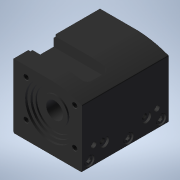
# Autodesk Inventor part: EGC-80-TB-KF___(0_0_Deckel RE)
Saved by Autodesk Inventor 2021 (Build 250183000, 183)
## iProperties
Created: 2026-04-25
Part Number: EGC-80-TB-KF___(0_0_Deckel RE)
Material: Generic
Catalog Web Link: www.3dfindit.com
Description: EGC-RE-TB-Antriebsdeckel RE
Vendor: FESTO
Document SubType Name: Modeling
Designer: psAdmin
Manufacturer: FESTO
Mass: 244.386 g
Surface Area: 426.779 cm^2
Volume: 244.386 cm^3
Density: 1 g/cm^3
Appearance: PSOLRGB-176-176-176
Category: PARTsolutions
Company: FESTO
Title: EGC-80-TB-KF___(0_0_Deckel RE)
Author: Cadenas PARTsolutions
Comments: Antriebsdeckel RE
PSOL_IDENT_0: {$CADENAS_DATA/23d-libs/festo/parts/e/egc/parts/egc_tb_deckel_re.prj},221 {VTYP=3D},{NB=EGC-80-TB-KF
PSOL_IDENT_1: ___(0_0_Deckel RE)},{LINA=EGC-80-TB-KF___(0_0_Deckel RE)},{NN=EGC-RE-TB},{DATE=12.11.2020 08:38:39},
PSOL_IDENT_2: {GEOMDATE=30.04.2020 12:28:00},{VERSION=},{LINEID=30},{WBVAR=ZUBA,ZUBC},{WBNUMERIC=ZUBA,ZUBC}  {NB=E
PSOL_IDENT_3: GC-80-TB-KF___(0_0_Deckel RE)},{LINA=EGC-80-TB-KF___(0_0_Deckel RE)},{KT=DUMMY},{TYP=EGC-80-TB-KF},{
PSOL_IDENT_4: VERS=3.000},{SIZE=80.000},{ZUBA=0},{ZUBC=0},{D1=48},{D2=16},{D3=46.5},{D4=25},{T1=2.1},{T2=27.0},{T4=
PSOL_IDENT_5: 4.00}
NB: EGC-80-TB-KF___(0_0_Deckel RE)
NN: EGC-RE-TB
NT: Antriebsdeckel RE
NBSYN: $TYP.___($ZUBA._$ZUBC._Deckel RE)
LINA: EGC-80-TB-KF___(0_0_Deckel RE)
CATALOG: Festo
TYP: EGC-80-TB-KF
VERS: 3
SIZE: 80
ZUBA: 0
ZUBC: 0
D1: 48
D2: 16
D3: 46.5
D4: 25
T1: 2.1
T2: 27
T4: 4
SUPPLIER: FESTO
ARTICLENO: EGC-80-TB-KF___(0_0_Deckel RE)
BOMINFO: EGC-80-TB-KF___(0_0_Deckel RE)
CREATOR: CADENAS GmbH
Autodesk Inventor part; units mm, degrees
sketch "Sketch_28" plane through (0, 0, 0) normal (0, 0, 1) x (1, 0, 0)
  line L0 (0, 61) -> (0, 0)
  line L1 (0, 0) -> (65, 0)
  line L2 (65, 0) -> (65, 55)
  arc A0 (65, 55) -> (36.5, 61) centre (32.036, -30.8916) ccw
  line L3 (36.5, 61) -> (0, 61)
  constraints: 8 end point, 2 point on circle, 1 centre point
extrude "Extrusion1" add sketch "Sketch_28" along normal blind 82
sketch "Sketch_20" plane through (0, 0, 0) normal (0, 0, 1) x (1, 0, 0)
  line L0 (-2, 5) -> (-2, -1)
  line L1 (-2, -1) -> (66, -1)
  line L2 (66, -1) -> (66, 57)
  line L3 (66, 57) -> (64, 57)
  line L4 (64, 57) -> (64, 55.4781)
  arc A0 (64.4301, 55.2752) -> (64, 55.4781) centre (38.6219, 1.1094) ccw
  arc A1 (65, 54.3725) -> (64.4301, 55.2752) centre (64, 54.3725) ccw
  line L5 (65, 54.3725) -> (65, 1)
  arc A2 (64, 0) -> (65, 1) centre (64, 1) ccw
  line L6 (64, 0) -> (1, 0)
  arc A3 (0, 1) -> (1, 0) centre (1, 1) ccw
  line L7 (0, 1) -> (0, 5)
  line L8 (0, 5) -> (-2, 5)
  constraints: 18 end point, 8 point on circle, 4 centre point
extrude "Extrusion2" cut sketch "Sketch_20" along normal blind 82
sketch "Sketch3" plane through (0, 0, 82) normal (0, 0, 1) x (1, 0, 0)
  point P0 (12, 16.5)
hole "Hole1" at (12, 16.5, 82) direction (0, 0, -1) diameter 4.134 depth 13 tip angle 120 countersink diameter 5 countersink angle 90 thread size "M5x0.8" class "6H" standard "ISO Metric profile"
sketch "Sketch4" plane through (0, 0, 82) normal (0, 0, 1) x (1, 0, 0)
  point P0 (12, 51.5)
hole "Hole2" at (12, 51.5, 82) direction (0, 0, -1) diameter 4.134 depth 13 tip angle 120 countersink diameter 5 countersink angle 90 thread size "M5x0.8" class "6H" standard "ISO Metric profile"
sketch "Sketch5" plane through (0, 0, 0) normal (0, 0, -1) x (-1, 0, 0)
  point P0 (-12, 16.5)
hole "Hole3" at (12, 16.5, 0) direction (0, 0, 1) diameter 4.134 depth 13 tip angle 120 countersink diameter 5 countersink angle 90 thread size "M5x0.8" class "6H" standard "ISO Metric profile"
sketch "Sketch6" plane through (0, 0, 0) normal (0, 0, -1) x (-1, 0, 0)
  point P0 (-12, 51.5)
hole "Hole4" at (12, 51.5, 0) direction (0, 0, 1) diameter 4.134 depth 13 tip angle 120 countersink diameter 5 countersink angle 90 thread size "M5x0.8" class "6H" standard "ISO Metric profile"
sketch "Sketch7" plane through (0, 0, 82) normal (0, 0, 1) x (1, 0, 0)
  point P0 (58, 16.5)
hole "Hole5" at (58, 16.5, 82) direction (0, 0, -1) diameter 4.134 depth 13 tip angle 120 countersink diameter 5 countersink angle 90 thread size "M5x0.8" class "6H" standard "ISO Metric profile"
sketch "Sketch8" plane through (0, 0, 82) normal (0, 0, 1) x (1, 0, 0)
  point P0 (58, 51.5)
hole "Hole6" at (58, 51.5, 82) direction (0, 0, -1) diameter 4.134 depth 13 tip angle 120 countersink diameter 5 countersink angle 90 thread size "M5x0.8" class "6H" standard "ISO Metric profile"
sketch "Sketch9" plane through (0, 0, 0) normal (0, 0, -1) x (-1, 0, 0)
  point P0 (-58, 16.5)
hole "Hole7" at (58, 16.5, 0) direction (0, 0, 1) diameter 4.134 depth 13 tip angle 120 countersink diameter 5 countersink angle 90 thread size "M5x0.8" class "6H" standard "ISO Metric profile"
sketch "Sketch10" plane through (0, 0, 0) normal (0, 0, -1) x (-1, 0, 0)
  point P0 (-58, 51.5)
hole "Hole8" at (58, 51.5, 0) direction (0, 0, 1) diameter 4.134 depth 13 tip angle 120 countersink diameter 5 countersink angle 90 thread size "M5x0.8" class "6H" standard "ISO Metric profile"
sketch "Sketch_13" plane through (0, 0, 0) normal (1, 0, 0) x (0, 1, 0)
  circle A0 centre (55.5, 71) radius 2.85
  constraints: 1 centre point
extrude "Extrusion3" add sketch "Sketch_13" against normal blind 2
sketch "Sketch12" plane through (65, 1, 0) normal (1, 0, 0) x (0, 0, -1)
  point P0 (-71, 16)
hole "Hole9" at (65, 17, 71) direction (-1, 0, 0) diameter 5 depth 3.1
sketch "Sketch13" plane through (65, 1, 0) normal (1, 0, 0) x (0, 0, -1)
  point P0 (-11, 16)
hole "Hole10" at (65, 17, 11) direction (-1, 0, 0) diameter 5 depth 3.1
sketch "Sketch_18" plane through (0, 14.5, 0) normal (0, 1, 0) x (1, 0, 0)
  line L0 (65, -61) -> (50.7066, -61)
  line L1 (50.7066, -61) -> (51.9, -58.933)
  line L2 (51.9, -58.933) -> (62.467, -58.933)
  line L3 (62.467, -58.933) -> (62.9, -58.5)
  line L4 (62.9, -58.5) -> (62.9, -56.5)
  line L5 (62.9, -56.5) -> (65, -56.5)
  line L6 (65, -56.5) -> (65, -61)
  line L7 (65, -61) -> (50.7066, -61)
  constraints: 16 end point
revolve "Revolution1" cut sketch "Sketch_18" angle 360 about axis through (65, 14.5, 61) along (1, 0, 0)
thread "Thread1" size "M5x0.8" class "6H" standard "ISO Metric profile" length 7.567
sketch "Sketch_19" plane through (0, 14.5, 0) normal (0, 1, 0) x (1, 0, 0)
  line L0 (65, -21) -> (50.7066, -21)
  line L1 (50.7066, -21) -> (51.9, -18.933)
  line L2 (51.9, -18.933) -> (62.467, -18.933)
  line L3 (62.467, -18.933) -> (62.9, -18.5)
  line L4 (62.9, -18.5) -> (62.9, -16.5)
  line L5 (62.9, -16.5) -> (65, -16.5)
  line L6 (65, -16.5) -> (65, -21)
  line L7 (65, -21) -> (50.7066, -21)
  constraints: 16 end point
revolve "Revolution2" cut sketch "Sketch_19" angle 360 about axis through (65, 14.5, 21) along (1, 0, 0)
thread "Thread2" size "M5x0.8" class "6H" standard "ISO Metric profile" length 7.567
sketch "Sketch_26" plane through (0, 6, 0) normal (0, 1, 0) x (1, 0, 0)
  line L0 (65, -7) -> (61.9, -7)
  line L1 (61.9, -7) -> (64.3, -4.6)
  line L2 (64.3, -4.6) -> (64.3, -3.25)
  line L3 (64.3, -3.25) -> (63.8, -2.75)
  line L4 (63.8, -2.75) -> (59.3, -2.75)
  line L5 (59.3, -2.75) -> (59.3, -2.25)
  line L6 (59.3, -2.25) -> (65, -2.25)
  line L7 (65, -2.25) -> (65, -7)
  line L8 (65, -7) -> (61.9, -7)
  constraints: 18 end point
revolve "Revolution3" cut sketch "Sketch_26" angle 360 about axis through (65, 6, 7) along (1, 0, 0)
sketch "Pattern_1_SKETCH_1" plane through (0, 6, 0) normal (0, 1, 0) x (1, 0, 0)
  line L0 (65, -38) -> (61.9, -38)
  line L1 (61.9, -38) -> (64.3, -35.6)
  line L2 (64.3, -35.6) -> (64.3, -34.25)
  line L3 (64.3, -34.25) -> (63.8, -33.75)
  line L4 (63.8, -33.75) -> (59.3, -33.75)
  line L5 (59.3, -33.75) -> (59.3, -33.25)
  line L6 (59.3, -33.25) -> (65, -33.25)
  line L7 (65, -33.25) -> (65, -38)
  line L8 (65, -38) -> (61.9, -38)
  constraints: 18 end point
sketch "Pattern_1_SKETCH_2" plane through (0, 6, 0) normal (0, 1, 0) x (1, 0, 0)
  line L0 (65, -75) -> (61.9, -75)
  line L1 (61.9, -75) -> (64.3, -72.6)
  line L2 (64.3, -72.6) -> (64.3, -71.25)
  line L3 (64.3, -71.25) -> (63.8, -70.75)
  line L4 (63.8, -70.75) -> (59.3, -70.75)
  line L5 (59.3, -70.75) -> (59.3, -70.25)
  line L6 (59.3, -70.25) -> (65, -70.25)
  line L7 (65, -70.25) -> (65, -75)
  line L8 (65, -75) -> (61.9, -75)
  constraints: 18 end point
revolve "Revolution4" cut sketch "Pattern_1_SKETCH_1" angle 360 about axis through (65, 6, 38) along (1, 0, 0)
revolve "Revolution5" cut sketch "Pattern_1_SKETCH_2" angle 360 about axis through (65, 6, 75) along (1, 0, 0)
sketch "Sketch_30" plane through (65, 0, 0) normal (1, 0, 0) x (0, 0, -1)
  line L0 (-9, 4.8453) -> (-7, 3.6906)
  line L1 (-7, 3.6906) -> (-5, 4.8453)
  line L2 (-5, 4.8453) -> (-5, 7.1547)
  line L3 (-5, 7.1547) -> (-7, 8.3094)
  line L4 (-7, 8.3094) -> (-9, 7.1547)
  line L5 (-9, 7.1547) -> (-9, 4.8453)
  constraints: 12 end point
extrude "Extrusion4" cut sketch "Sketch_30" against normal blind 3.2
sketch "Pattern_2_SKETCH_1" plane through (65, 0, 0) normal (1, 0, 0) x (0, 0, -1)
  line L0 (-40, 4.8453) -> (-38, 3.6906)
  line L1 (-38, 3.6906) -> (-36, 4.8453)
  line L2 (-36, 4.8453) -> (-36, 7.1547)
  line L3 (-36, 7.1547) -> (-38, 8.3094)
  line L4 (-38, 8.3094) -> (-40, 7.1547)
  line L5 (-40, 7.1547) -> (-40, 4.8453)
  constraints: 12 end point
sketch "Pattern_2_SKETCH_2" plane through (65, 0, 0) normal (1, 0, 0) x (0, 0, -1)
  line L0 (-77, 4.8453) -> (-75, 3.6906)
  line L1 (-75, 3.6906) -> (-73, 4.8453)
  line L2 (-73, 4.8453) -> (-73, 7.1547)
  line L3 (-73, 7.1547) -> (-75, 8.3094)
  line L4 (-75, 8.3094) -> (-77, 7.1547)
  line L5 (-77, 7.1547) -> (-77, 4.8453)
  constraints: 12 end point
extrude "Extrusion5" cut sketch "Pattern_2_SKETCH_1" against normal blind 3.2
extrude "Extrusion6" cut sketch "Pattern_2_SKETCH_2" against normal blind 3.2
sketch "Sketch_27" plane through (0, 51.7, 0) normal (0, 1, 0) x (1, 0, 0)
  line L0 (0, -44) -> (0, -66)
  line L1 (0, -66) -> (48, -66)
  arc A0 (48, -66) -> (53, -61) centre (48, -61) ccw
  line L2 (53, -61) -> (53, -49)
  arc A1 (53, -49) -> (48, -44) centre (48, -49) ccw
  line L3 (48, -44) -> (0, -44)
  constraints: 8 end point, 4 point on circle, 2 centre point
extrude "Extrusion7" cut sketch "Sketch_27" along normal blind 9.3
sketch "Sketch_24" plane through (0, 0, 0) normal (1, 0, 0) x (0, 1, 0)
  line L0 (59.05, 68) -> (59.05, 42)
  line L1 (59.05, 42) -> (61, 42)
  line L2 (61, 42) -> (61, 68)
  line L3 (61, 68) -> (59.05, 68)
  constraints: 8 end point
extrude "Extrusion8" cut sketch "Sketch_24" along normal blind 2
sketch "Sketch_32" plane through (35, 0, 0) normal (1, 0, 0) x (0, 0, -1)
  line L0 (0, 34) -> (-82, 34)
  line L1 (-82, 34) -> (-82, 58)
  line L2 (-82, 58) -> (-79.9, 58)
  line L3 (-79.9, 58) -> (-79.9, 55)
  line L4 (-79.9, 55) -> (-78, 55)
  line L5 (-78, 55) -> (-78, 52.15)
  line L6 (-78, 52.15) -> (-76.65, 52.15)
  line L7 (-76.65, 52.15) -> (-76.65, 46.5)
  line L8 (-76.65, 46.5) -> (-78, 46.5)
  line L9 (-78, 46.5) -> (-78, 42)
  line L10 (-78, 42) -> (-51, 42)
  line L11 (-51, 42) -> (-51, 42.8)
  line L12 (-51, 42.8) -> (-31, 42.8)
  line L13 (-31, 42.8) -> (-31, 42)
  line L14 (-31, 42) -> (-4, 42)
  line L15 (-4, 42) -> (-4, 46.5)
  line L16 (-4, 46.5) -> (-31, 46.5)
  line L17 (-31, 46.5) -> (-31, 57.25)
  line L18 (-31, 57.25) -> (-2.1, 57.25)
  line L19 (-2.1, 57.25) -> (-2.1, 58)
  line L20 (-2.1, 58) -> (0, 58)
  line L21 (0, 58) -> (0, 34)
  line L22 (0, 34) -> (-82, 34)
  constraints: 46 end point
revolve "Revolution6" cut sketch "Sketch_32" angle 360 about axis through (35, 34, 0) along (0, 0, -1)
ref_plane "AXIAL_R_H_XY" through (35, 34, 0) normal (0, 0, 1) x (1, 0, 0)
ref_plane "AXIAL_R_H_YZ" through (35, 34, 0) normal (1, 0, 0) x (0, 1, 0)
ref_plane "AXIAL_R_H_ZX" through (35, 34, 0) normal (0, 1, 0) x (0, 0, 1)
ref_plane "AXIAL_R_V_XY" through (35, 34, 82) normal (0, 0, -1) x (1, 0, 0)
ref_plane "AXIAL_R_V_YZ" through (35, 34, 82) normal (1, 0, 0) x (0, -1, 0)
ref_plane "AXIAL_R_V_ZX" through (35, 34, 82) normal (0, -1, 0) x (0, 0, -1)
ref_plane "CUP1_XY" through (35, 34, 0) normal (0, 0, -1) x (1, 0, 0)
ref_plane "CUP1_YZ" through (35, 34, 0) normal (1, 0, 0) x (0, -1, 0)
ref_plane "CUP1_ZX" through (35, 34, 0) normal (0, -1, 0) x (0, 0, -1)
ref_plane "CUP2_XY" through (35, 34, 82) normal (0, 0, 1) x (1, 0, 0)
ref_plane "CUP2_YZ" through (35, 34, 82) normal (1, 0, 0) x (0, 1, 0)
ref_plane "CUP2_ZX" through (35, 34, 82) normal (0, 1, 0) x (0, 0, 1)
ref_plane "DR_XY" through (0, -0.5, 41) normal (-1, 0, 0) x (0, 0, 1)
ref_plane "DR_YZ" through (0, -0.5, 41) normal (0, 0, 1) x (0, 1, 0)
ref_plane "DR_ZX" through (0, -0.5, 41) normal (0, 1, 0) x (-1, 0, 0)
ref_plane "TO_AK_XY" through (0, 51.7, 55) normal (1, 0, 0) x (0, 0, -1)
ref_plane "TO_AK_YZ" through (0, 51.7, 55) normal (0, 0, -1) x (0, 1, 0)
ref_plane "TO_AK_ZX" through (0, 51.7, 55) normal (0, 1, 0) x (1, 0, 0)
ref_plane "WELLENZAPFEN_R_H_XY" through (35, 34, 4) normal (0, 0, 1) x (1, 0, 0)
ref_plane "WELLENZAPFEN_R_H_YZ" through (35, 34, 4) normal (1, 0, 0) x (0, 1, 0)
ref_plane "WELLENZAPFEN_R_H_ZX" through (35, 34, 4) normal (0, 1, 0) x (0, 0, 1)
ref_plane "WELLENZAPFEN_R_V_XY" through (35, 34, 78) normal (0, 0, -1) x (1, 0, 0)
ref_plane "WELLENZAPFEN_R_V_YZ" through (35, 34, 78) normal (1, 0, 0) x (0, -1, 0)
ref_plane "WELLENZAPFEN_R_V_ZX" through (35, 34, 78) normal (0, -1, 0) x (0, 0, -1)
body "Solid1"
